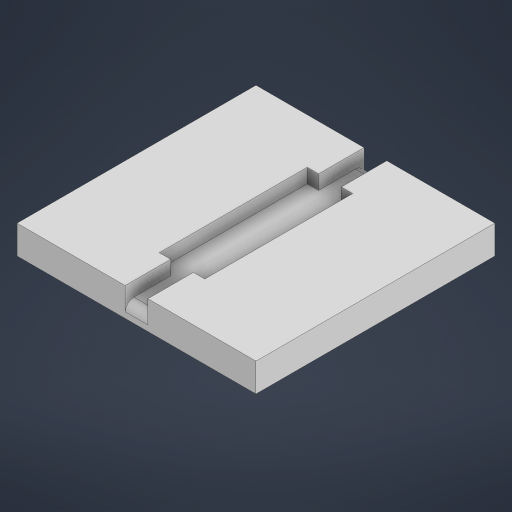
# Autodesk Inventor part: 09_centerlegg_topplate
Saved by Autodesk Inventor 2024 (Build 280153000, 153)
## iProperties
Created: 2023-05-24
Part Number: 09_centerlegg_topplate
Material: Generic
Document SubType Name: Modeling
Designer: aasmu
Density: 1 g/cm^3
Appearance: Default
Author: aasmu
Autodesk Inventor part; units mm, degrees
ref_plane "YZ Plane" through (0, 0, 0) normal (1, 0, 0) x (0, 1, 0)
ref_plane "XZ Plane" through (0, 0, 0) normal (0, 1, 0) x (-1, 0, 0)
ref_plane "XY Plane" through (0, 0, 0) normal (0, 0, 1) x (1, 0, 0)
sketch "Sketch1" plane through (0, 0, 0) normal (0, 1, 0) x (-1, 0, 0)
  line L0 (0, 0) -> (84, 0)
  line L1 (84, 0) -> (84, -84)
  line L2 (84, -84) -> (0, -84)
  line L3 (0, -84) -> (0, 0)
  line L4 (16, -16) -> (68, -16)
  line L5 (68, -16) -> (68, -68)
  line L6 (68, -68) -> (16, -68)
  line L7 (16, -68) -> (16, -16)
  line L8 (0, 0) -> (84, -84) construction
  line L9 (84, 0) -> (0, -84) construction
  line L10 (46, 0) -> (46, -16)
  line L11 (38, 0) -> (38, -16)
  line L12 (38, -68) -> (38, -84)
  line L13 (46, -68) -> (46, -84)
  line L14 (46, -76) -> (38, -76) construction
  line L15 (42, -76) -> (42, -68) construction
  line L16 (50, -16) -> (50, -68)
  line L17 (34, -68) -> (34, -16)
  dimension "d0" = 52
  dimension "d1" = 84
  dimension "d2" = 4
  dimension "d3" = 4
  dimension "d4" = 4
  constraints: 36 end point, 15 point on line, 8 perpendicular, 5 parallel, 4 midpoint, 2 collinear, 2 horizontal, 1 vertical
  measures "d0" distance of L4.start L4.end
  measures "d1" distance of L0.start L0.end
  measures "d2" distance from line of L15.start L13
  measures "d3" distance from line of L13.start L16
  measures "d4" distance from line of L12.start L17
extrude "Extrusion1" add sketch "Sketch1" along normal blind 10 contours L0 L11 L4 L7 L6 L12 L2 L3 | L0 L1 L2 L13 L6 L5 L4 L10 | L17 L6 L7 L4 | L4 L5 L6 L16
extrude "Extrusion2" add sketch "Sketch1" along normal blind 5 contours L0 L10 L4 L11 | L4 L16 L6 L17 | L12 L6 L13 L2
extrude "Extrusion3" add sketch "Sketch1" against normal blind 10 contours L4 L16 L6 L17 | L17 L6 L7 L4 | L4 L5 L6 L16
fillet "Fillet1" radius 2 4 edges at (-68, -10, -42) (-42, -10, -16) (-16, -10, -42) (-42, -10, -68)
fillet "Fillet2" radius 3 2 edges at (-42, 5, 0) (-42, 5, -84)
equation "\"d0\" = inner_carriage_length - 2 * inner_carriage_width"
equation "\"d1\" = long_centerlegg_width"
equation "\"d2\" = cabel_shaft_size"
equation "\"d3\" = cabel_shaft_size"
equation "\"d4\" = cabel_shaft_size"
equation "\"d5\" = 0.5 * centerlegg_topplate_thicknes"
equation "\"d7\" = 0.5 * centerlegg_topplate_thicknes - centerlegg_grove_depth"
equation "\"d9\" = 0.5 * centerlegg_topplate_thicknes"
equation "\"centerlegg_grove_depth\" = 5"
equation "\"inner_carriage_length\" = 72"
equation "\"inner_carriage_width\" = 10"
equation "\"long_centerlegg_width\" = 84"
equation "\"cabel_shaft_size\" = 4"
equation "\"centerlegg_topplate_thicknes\" = 20"
body "Solid1"
